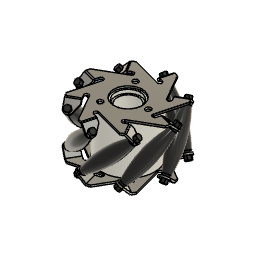
麦克纳姆轮A v5 (Autodesk Fusion 360 design; units mm, degrees)
Autodesk Fusion 360 part; units mm, degrees
note: some values were not read from the file. Set by a fixed rule: which sketch regions a step uses.
sketch "草图1" plane through (0, 0, 0) normal (0, 0, 1) x (1, 0, 0)
  circle A0 centre (0, 0) radius 8
  line L0 (-15.1925, 2.6566) -> (-15.1925, 19.6566)
  line L1 (-15.1925, 19.6566) -> (-10.2428, 14.7068)
  arc A1 (-10.2428, 14.7068) -> (-8.8643, 12.6212) centre (-9.5407, 13.6725) ccw
  line L2 (-12.6212, -8.8643) -> (-24.642, 3.1565)
  line L3 (-24.642, 3.1565) -> (-17.642, 3.1565)
  arc A2 (-17.642, 3.1565) -> (-15.1925, 2.6566) centre (-16.4142, 2.9216) ccw
  line L4 (-2.6566, -15.1925) -> (-19.6566, -15.1925)
  line L5 (-19.6566, -15.1925) -> (-14.7068, -10.2428)
  arc A3 (-14.7068, -10.2428) -> (-12.6212, -8.8643) centre (-13.6725, -9.5407) ccw
  line L6 (8.8643, -12.6212) -> (-3.1565, -24.642)
  line L7 (-3.1565, -24.642) -> (-3.1565, -17.642)
  arc A4 (-3.1565, -17.642) -> (-2.6566, -15.1925) centre (-2.9216, -16.4142) ccw
  line L8 (15.1925, -2.6566) -> (15.1925, -19.6566)
  line L9 (15.1925, -19.6566) -> (10.2428, -14.7068)
  arc A5 (10.2428, -14.7068) -> (8.8643, -12.6212) centre (9.5407, -13.6725) ccw
  line L10 (12.6212, 8.8643) -> (24.642, -3.1565)
  line L11 (24.642, -3.1565) -> (17.642, -3.1565)
  arc A6 (17.642, -3.1565) -> (15.1925, -2.6566) centre (16.4142, -2.9216) ccw
  line L12 (2.6566, 15.1925) -> (19.6566, 15.1925)
  line L13 (19.6566, 15.1925) -> (14.7068, 10.2428)
  arc A7 (14.7068, 10.2428) -> (12.6212, 8.8643) centre (13.6725, 9.5407) ccw
  line L14 (-8.8643, 12.6212) -> (3.1565, 24.642)
  line L15 (3.1565, 24.642) -> (3.1565, 17.642)
  arc A8 (3.1565, 17.642) -> (2.6566, 15.1925) centre (2.9216, 16.4142) ccw
  dimension "d1" = 16
  dimension "d2" = 2.5
  dimension "d3" = 45
  dimension "d4" = 7
  dimension "d5" = 17
  dimension "d7" = 360
  constraint coincident A0.centre origin
  constraint vertical L0
  constraint coincident L0 A2.end
  constraint coincident L12.start A8.end
  measures "d1" diameter of A0
  measures "d2" distance of L1.end A1.end
  measures "d3" angle of L0 L1
  measures "d4" distance of L0.end L1.end
  measures "d5" distance of L0.start L0.end
extrude "拉伸1" add sketch "草图1" along normal blind 1 makes body 1
sketch "草图2" plane through (0, 0, 1) normal (0, 0, 1) x (-1, 0, 0)
  circle A0 centre (0, 0) radius 8
  line L0 (-3.1565, -17.642) -> (-3.1565, -24.642)
  line L1 (-3.1565, -24.642) -> (8.8643, -12.6212)
  arc A1 (10.2428, -14.7068) -> (8.8643, -12.6212) centre (9.5407, -13.6725) ccw
  line L2 (10.2428, -14.7068) -> (15.1925, -19.6566)
  line L3 (15.1925, -19.6566) -> (15.1925, -2.6566)
  arc A2 (17.642, -3.1565) -> (15.1925, -2.6566) centre (16.4142, -2.9216) ccw
  line L4 (17.642, -3.1565) -> (24.642, -3.1565)
  line L5 (24.642, -3.1565) -> (12.6212, 8.8643)
  arc A3 (14.7068, 10.2428) -> (12.6212, 8.8643) centre (13.6725, 9.5407) ccw
  line L6 (14.7068, 10.2428) -> (19.6566, 15.1925)
  line L7 (19.6566, 15.1925) -> (2.6566, 15.1925)
  arc A4 (3.1565, 17.642) -> (2.6566, 15.1925) centre (2.9216, 16.4142) ccw
  line L8 (3.1565, 17.642) -> (3.1565, 24.642)
  line L9 (3.1565, 24.642) -> (-8.8643, 12.6212)
  arc A5 (-10.2428, 14.7068) -> (-8.8643, 12.6212) centre (-9.5407, 13.6725) ccw
  line L10 (-10.2428, 14.7068) -> (-15.1925, 19.6566)
  line L11 (-15.1925, 19.6566) -> (-15.1925, 2.6566)
  arc A6 (-17.642, 3.1565) -> (-15.1925, 2.6566) centre (-16.4142, 2.9216) ccw
  line L12 (-17.642, 3.1565) -> (-24.642, 3.1565)
  line L13 (-24.642, 3.1565) -> (-12.6212, -8.8643)
  arc A7 (-14.7068, -10.2428) -> (-12.6212, -8.8643) centre (-13.6725, -9.5407) ccw
  line L14 (-14.7068, -10.2428) -> (-19.6566, -15.1925)
  line L15 (-19.6566, -15.1925) -> (-2.6566, -15.1925)
  arc A8 (-3.1565, -17.642) -> (-2.6566, -15.1925) centre (-2.9216, -16.4142) ccw
  line L16 (3.1565, 17.642) -> (5.1565, 17.642)
  line L17 (5.1565, 17.642) -> (5.1565, 24.6526)
  line L18 (5.1565, 24.6526) -> (3.1565, 24.6526)
  line L19 (3.1565, 24.6526) -> (3.1565, 17.642)
  line L20 (-13.7858, 21.0782) -> (-15.2, 19.664)
  line L21 (-15.2, 19.664) -> (-10.2428, 14.7068)
  line L22 (-8.8286, 16.121) -> (-13.7858, 21.0782)
  line L23 (-10.2428, 14.7068) -> (-8.8286, 16.121)
  line L24 (-24.6526, 5.1565) -> (-24.6526, 3.1565)
  line L25 (-24.6526, 3.1565) -> (-17.642, 3.1565)
  line L26 (-17.642, 5.1565) -> (-24.6526, 5.1565)
  line L27 (-17.642, 3.1565) -> (-17.642, 5.1565)
  line L28 (-21.0782, -13.7858) -> (-19.664, -15.2)
  line L29 (-19.664, -15.2) -> (-14.7068, -10.2428)
  line L30 (-16.121, -8.8286) -> (-21.0782, -13.7858)
  line L31 (-14.7068, -10.2428) -> (-16.121, -8.8286)
  line L32 (-5.1565, -24.6526) -> (-3.1565, -24.6526)
  line L33 (-3.1565, -24.6526) -> (-3.1565, -17.642)
  line L34 (-5.1565, -17.642) -> (-5.1565, -24.6526)
  line L35 (-3.1565, -17.642) -> (-5.1565, -17.642)
  line L36 (13.7858, -21.0782) -> (15.2, -19.664)
  line L37 (15.2, -19.664) -> (10.2428, -14.7068)
  line L38 (8.8286, -16.121) -> (13.7858, -21.0782)
  line L39 (10.2428, -14.7068) -> (8.8286, -16.121)
  line L40 (24.6526, -5.1565) -> (24.6526, -3.1565)
  line L41 (24.6526, -3.1565) -> (17.642, -3.1565)
  line L42 (17.642, -5.1565) -> (24.6526, -5.1565)
  line L43 (17.642, -3.1565) -> (17.642, -5.1565)
  line L44 (21.0782, 13.7858) -> (19.664, 15.2)
  line L45 (19.664, 15.2) -> (14.7068, 10.2428)
  line L46 (16.121, 8.8286) -> (21.0782, 13.7858)
  line L47 (14.7068, 10.2428) -> (16.121, 8.8286)
  dimension "d10" = 2
  dimension "d12" = 360
  constraint horizontal L16
  constraint vertical L17
  constraint horizontal L18
  constraint vertical L19
  constraint coincident A4.start L8.start
  measures "d10" distance of L17.end L18.end
extrude "拉伸2" add sketch "草图2" against normal blind 1 contours L0 L32 L33 L34 L35 | L14 L28 L29 L30 L31 | L2 L36 L37 L38 L39 | L12 L24 L25 L26 L27 | L4 L40 L41 L42 L43 | L10 L20 L21 L22 L23 | L6 L44 L45 L46 L47 | L8 L16 L17 L18 L19 bodies 1
sketch "草图3" plane through (0, 0, 1) normal (0, 0, 1) x (-1, 0, 0)
  circle A0 centre (0, 0) radius 8
  line L0 (-3.1565, -24.642) -> (8.8643, -12.6212)
  arc A1 (10.2428, -14.7068) -> (8.8643, -12.6212) centre (9.5407, -13.6725) ccw
  line L1 (10.2428, -14.7068) -> (8.8286, -16.121)
  line L2 (8.8286, -16.121) -> (13.7858, -21.0782)
  line L3 (13.7858, -21.0782) -> (15.2, -19.664)
  line L4 (15.2, -19.664) -> (15.1925, -19.6566)
  line L5 (15.1925, -19.6566) -> (15.1925, -2.6566)
  arc A2 (17.642, -3.1565) -> (15.1925, -2.6566) centre (16.4142, -2.9216) ccw
  line L6 (17.642, -3.1565) -> (17.642, -5.1565)
  line L7 (17.642, -5.1565) -> (24.6526, -5.1565)
  line L8 (24.6526, -5.1565) -> (24.6526, -3.1565)
  line L9 (24.6526, -3.1565) -> (24.642, -3.1565)
  line L10 (24.642, -3.1565) -> (12.6212, 8.8643)
  arc A3 (14.7068, 10.2428) -> (12.6212, 8.8643) centre (13.6725, 9.5407) ccw
  line L11 (14.7068, 10.2428) -> (16.121, 8.8286)
  line L12 (16.121, 8.8286) -> (21.0782, 13.7858)
  line L13 (21.0782, 13.7858) -> (19.664, 15.2)
  line L14 (19.664, 15.2) -> (19.6566, 15.1925)
  line L15 (19.6566, 15.1925) -> (2.6566, 15.1925)
  arc A4 (3.1565, 17.642) -> (2.6566, 15.1925) centre (2.9216, 16.4142) ccw
  line L16 (3.1565, 17.642) -> (5.1565, 17.642)
  line L17 (5.1565, 17.642) -> (5.1565, 24.6526)
  line L18 (5.1565, 24.6526) -> (3.1565, 24.6526)
  line L19 (3.1565, 24.6526) -> (3.1565, 24.642)
  line L20 (3.1565, 24.642) -> (-8.8643, 12.6212)
  arc A5 (-10.2428, 14.7068) -> (-8.8643, 12.6212) centre (-9.5407, 13.6725) ccw
  line L21 (-10.2428, 14.7068) -> (-8.8286, 16.121)
  line L22 (-8.8286, 16.121) -> (-13.7858, 21.0782)
  line L23 (-13.7858, 21.0782) -> (-15.2, 19.664)
  line L24 (-15.2, 19.664) -> (-15.1925, 19.6566)
  line L25 (-15.1925, 19.6566) -> (-15.1925, 2.6566)
  arc A6 (-17.642, 3.1565) -> (-15.1925, 2.6566) centre (-16.4142, 2.9216) ccw
  line L26 (-17.642, 3.1565) -> (-17.642, 5.1565)
  line L27 (-17.642, 5.1565) -> (-24.6526, 5.1565)
  line L28 (-24.6526, 5.1565) -> (-24.6526, 3.1565)
  line L29 (-24.6526, 3.1565) -> (-24.642, 3.1565)
  line L30 (-24.642, 3.1565) -> (-12.6212, -8.8643)
  arc A7 (-14.7068, -10.2428) -> (-12.6212, -8.8643) centre (-13.6725, -9.5407) ccw
  line L31 (-14.7068, -10.2428) -> (-16.121, -8.8286)
  line L32 (-16.121, -8.8286) -> (-21.0782, -13.7858)
  line L33 (-21.0782, -13.7858) -> (-19.664, -15.2)
  line L34 (-19.664, -15.2) -> (-19.6566, -15.1925)
  line L35 (-19.6566, -15.1925) -> (-2.6566, -15.1925)
  arc A8 (-3.1565, -17.642) -> (-2.6566, -15.1925) centre (-2.9216, -16.4142) ccw
  line L36 (-3.1565, -17.642) -> (-5.1565, -17.642)
  line L37 (-5.1565, -17.642) -> (-5.1565, -24.6526)
  line L38 (-5.1565, -24.6526) -> (-3.1565, -24.6526)
  line L39 (-3.1565, -24.6526) -> (-3.1565, -24.642)
  circle A9 centre (0, 0) radius 11.5 construction
  line L40 (-14, 0) -> (17, 0)
  circle A10 centre (11.5, 0) radius 1.5
  circle A11 centre (-5.75, 9.9593) radius 1.5
  circle A12 centre (-5.75, -9.9593) radius 1.5
  dimension "d15" = 23
  dimension "d16" = 3
  dimension "d18" = 360
  constraint coincident A0.centre A9.centre
  constraint horizontal L40
  constraint coincident A9 A10.centre
  constraint coincident L40 A10.centre
  constraint coincident A0.centre L40
  measures "d15" diameter of A9
  measures "d16" diameter of A10
extrude "拉伸3" cut sketch "草图3" against normal blind 1 contours L40 A10 | L40 A10 | A11 | A12 bodies 1
sketch "草图4" plane through (-24.6526, 0, 0) normal (-1, 0, 0) x (0, -1, 0)
  line L0 (-3.1565, 1) -> (-5.1565, 1)
  line L1 (-5.1565, 1) -> (-5.1565, 0)
  line L2 (-5.1565, 0) -> (-3.1565, 0)
  line L3 (-3.1565, 0) -> (-3.1565, 1)
  line L4 (-3.1565, 0) -> (-5.1565, 0)
  line L5 (-5.1565, 0) -> (-5.1565, 1)
  line L6 (-12.9208, 0.5) -> (-0.2781, 0.5)
  line L7 (-10.8134, 5.2426) -> (-5.8636, 0.2929)
  arc A0 (-5.8636, 0.2929) -> (-5.1565, 0) centre (-5.0451, 1.2689) ccw
  line L8 (-5.1565, 1) -> (-10.1063, 5.9497)
  line L9 (-10.1063, 5.9497) -> (-10.8134, 5.2426)
  line L10 (-2.6566, 0) -> (-19.6566, 0)
  dimension "d82" = 1
  dimension "d83" = 7
  dimension "d84" = 7
  dimension "d85" = 45
  constraint coincident L2.end L3.start
  constraint coincident L1.end L2.start
  constraint coincident L0.end L1.start
  constraint symmetric L1.end L6 L0.end
  constraint symmetric L0.end L6 L1.end
  constraint perpendicular L7 L9
  constraint perpendicular L8 L9
  constraint parallel L6 L10
  measures "d82" distance of L7.start L8.end
  measures "d83" distance of L7.start L7.end
  measures "d84" distance of L0.end L8.end
  measures "d85" angle of L6 L8
extrude "拉伸4" add sketch "草图4" against normal blind 7 contours L0 L1 L3 L5 L6 bodies 1
extrude "拉伸17" add sketch "草图4" against normal blind 7 contours L1 L5 L6 L7 L8 L9 | L1 L5 L6 L7 A0 bodies 1
sketch "草图22" plane through (0, 2.0783, -2.0783) normal (0, -0.707107, 0.707107) x (1, 0, 0)
  line L0 (-24.6526, 11.3533) -> (-24.6526, 4.3533)
  line L1 (-24.6526, 4.3533) -> (-17.6526, 4.3533)
  line L2 (-17.6526, 4.3533) -> (-17.6526, 11.3533)
  line L3 (-17.6526, 11.3533) -> (-24.6526, 11.3533)
  line L4 (-17.6526, 6.3533) -> (-21.1526, 11.3533)
  dimension "d88" = 2
  constraint coincident L2 L4.start
  constraint midpoint L3 L4.end
  measures "d88" distance of L1.end L4.start
sketch "草图23" plane through (-19.4026, 8.3385, 4.182) normal (0, -0.707107, 0.707107) x (1, 0, 0)
extrude "拉伸18" cut sketch "草图22" against normal blind 1 contours L2 L3 L4 bodies 1
sketch "草图24" plane through (0, 2.0783, -2.0783) normal (0, -0.707107, 0.707107) x (1, 0, 0)
  line L0 (-17.6526, 6.3533) -> (-21.1526, 11.3533)
  line L1 (-21.1526, 11.3533) -> (-24.6526, 11.3533)
  line L2 (-24.6526, 11.3533) -> (-24.6526, 4.3533)
  line L3 (-24.6526, 4.3533) -> (-17.6526, 4.3533)
  line L4 (-17.6526, 4.3533) -> (-17.6526, 6.3533)
  line L5 (-20.4654, 10.3716) -> (-21.1526, 11.3533)
  line L6 (-24.6526, 11.3533) -> (-24.6526, 9.0517)
  arc A0 (-20.4654, 10.3716) -> (-24.6526, 9.0517) centre (-22.3509, 9.0517) ccw
  constraint tangent L0 A0
  constraint tangent L1 A0
  constraint tangent L2 A0
  constraint coincident L0.end L1.start
  constraint tangent L5 A0
  constraint coincident L1.end L2.start
  constraint coincident L2 L6.end
extrude "拉伸19" cut sketch "草图24" against normal blind 1 contours L0 L1 L5 A0 | L1 L2 L6 A0 bodies 1
sketch "草图25" plane through (0, 2.0783, -2.0783) normal (0, -0.707107, 0.707107) x (1, 0, 0)
  arc A0 (-20.4654, 10.3716) -> (-24.6526, 9.0517) centre (-22.3509, 9.0517) ccw
  line L0 (-24.6526, 9.0517) -> (-24.6526, 4.3533)
  line L1 (-24.6526, 4.3533) -> (-17.6526, 4.3533)
  line L2 (-17.6526, 4.3533) -> (-17.6526, 6.3533)
  line L3 (-17.6526, 6.3533) -> (-20.4654, 10.3716)
  circle A1 centre (-22.3509, 9.0517) radius 1.5
  dimension "d93" = 3
  constraint concentric A0 A1
  measures "d93" diameter of A1
extrude "拉伸20" cut sketch "草图25" against normal blind 1 contours A1 bodies 1
pattern_circular "C-阵列3" count 8 over 360 about axis through (0, 0, 1.75) along (0, 0, 1) of "拉伸17", "拉伸18", "拉伸19", "拉伸20"
copy_body "实体->零部件12" bodies 1 removing the originals makes body 2 in component "Component'"
sketch "草图26" plane through (0, 0, 0) normal (0, 0, 1) x (1, 0, 0)
  circle A0 centre (0, 0) radius 15
  dimension "d98" = 30
  constraint coincident A0.centre origin
  measures "d98" diameter of A0
extrude "拉伸21" add sketch "草图26" along normal blind 28 separate body makes body 3
sketch "草图27" plane through (0, 0, 28) normal (0, 0, 1) x (-1, 0, 0)
  circle A0 centre (0, 0) radius 15
  circle A1 centre (0, 0) radius 6
  dimension "d101" = 12
  constraint coincident A0.centre A1.centre
  measures "d101" diameter of A1
extrude "拉伸22" cut sketch "草图27" against normal blind 30 contours A1 bodies 3
sketch "草图28" plane through (0, 0, 28) normal (0, 0, 1) x (-1, 0, 0)
  circle A0 centre (0, 0) radius 6
  circle A1 centre (0, 0) radius 15
  circle A2 centre (0, 0) radius 7
  dimension "d104" = 14
  constraint coincident A0.centre A1.centre
  measures "d104" diameter of A2
extrude "拉伸23" cut sketch "草图28" against normal blind 2 contours A0 | A2 bodies 3
sketch "草图29" plane through (0, 0, 0) normal (0, 0, -1) x (1, 0, 0)
  circle A0 centre (0, 0) radius 6
  circle A1 centre (0, 0) radius 15
  circle A2 centre (0, 0) radius 7
  dimension "d107" = 14
  constraint concentric A0 A2
  measures "d107" diameter of A2
extrude "拉伸24" cut sketch "草图29" against normal blind 2 contours A0 | A2 bodies 3
sketch "草图30" plane through (0, 0, 28) normal (0, 0, 1) x (-1, 0, 0)
  circle A0 centre (0, 0) radius 7
  circle A1 centre (0, 0) radius 15
  circle A2 centre (0, 0) radius 11.5 construction
  line L0 (14, 0) -> (-14, 0)
  circle A3 centre (-11.5, 0) radius 1.5
  circle A4 centre (5.75, -9.9593) radius 1.5
  circle A5 centre (5.75, 9.9593) radius 1.5
  dimension "d110" = 23
  dimension "d111" = 3
  dimension "d113" = 360
  constraint coincident A0.centre A1.centre
  constraint horizontal L0
  constraint coincident A2 A3.centre
  constraint coincident L0 A3.centre
  constraint coincident A0.centre L0
  measures "d110" diameter of A2
  measures "d111" diameter of A3
extrude "拉伸25" cut sketch "草图30" against normal blind 30 contours L0 A3 | L0 A3 | A4 | A5 bodies 3
copy_body "实体->零部件13" bodies 3 removing the originals makes body 4 in component "Component''"
ref_plane "工作平面5" through (-22.2607, 1.3506, 3.3237) normal (0.183013, -0.683013, 0.707107) x (0.183013, -0.683013, -0.707107)
ref_plane "工作平面6" through (-14.7856, -16.6957, 24.6763) normal (-0.353553, 0.612372, -0.707107) x (-0.353553, 0.612372, 0.707107)
sketch "草图31" plane through (-14.7856, -16.6957, 24.6763) normal (-0.353553, 0.612372, -0.707107) x (-0.353553, 0.612372, 0.707107)
  circle A0 centre (-0.9979, -1.1984) radius 1.5
  arc A1 (-2.3178, 0.6872) -> (-0.9979, -3.5) centre (-0.9979, -1.1984) ccw
  line L0 (-0.9979, -3.5) -> (3.7005, -3.5)
  line L1 (3.7005, -3.5) -> (3.7005, 3.5)
  line L2 (3.7005, 3.5) -> (1.7005, 3.5)
  line L3 (1.7005, 3.5) -> (-2.3178, 0.6872)
  circle A2 centre (-0.9979, -1.1984) radius 2
  dimension "d126" = 4
  constraint concentric A0 A2
  measures "d126" diameter of A2
sketch "草图32" plane through (-22.2607, 1.3506, 3.3237) normal (0.183013, -0.683013, 0.707107) x (0.183013, -0.683013, -0.707107)
  circle A0 centre (-0.9979, -1.1984) radius 1.5
  arc A1 (-2.3178, 0.6872) -> (-0.9979, -3.5) centre (-0.9979, -1.1984) ccw
  line L0 (-0.9979, -3.5) -> (3.7005, -3.5)
  line L1 (3.7005, -3.5) -> (3.7005, 3.5)
  line L2 (3.7005, 3.5) -> (1.7005, 3.5)
  line L3 (1.7005, 3.5) -> (-2.3178, 0.6872)
  circle A2 centre (-0.9979, -1.1984) radius 2
  dimension "d127" = 4
  constraint concentric A0 A2
  measures "d127" diameter of A2
ref_plane "工作平面7" through (-18.983, -8.3097, 13.5908) normal (0.269433, -0.650469, 0.710138) x (0.184952, -0.688729, -0.701032)
sketch "草图33" plane through (-18.983, -8.3097, 13.5908) normal (0.269433, -0.650469, 0.710138) x (0.184952, -0.688729, -0.701032)
  circle A0 centre (-0.5, -0.5) radius 4
  dimension "d128" = 8
  measures "d128" diameter of A0
loft "放样2" add profiles "草图32", "草图33", "草图31" section 1 contours A2 section 2 section 3 contours A2 separate body makes body 5
sketch "草图34" plane through (-0.4843, 1.8074, -1.8712) normal (-0.183013, 0.683013, -0.707107) x (-0.965926, -0.258819, 0)
  circle A0 centre (22.3509, 8.3446) radius 2
  circle A1 centre (22.3509, 8.3446) radius 1.5
  dimension "d129" = 3
  constraint concentric A0 A1
  measures "d129" diameter of A1
extrude "拉伸26" add sketch "草图34" along normal blind 4 contours A1 bodies 5
sketch "草图35" plane through (7.9356, -13.7448, 15.8712) normal (0.353553, -0.612372, 0.707107) x (0.866025, 0.5, 0)
  circle A0 centre (-22.3509, 11.4544) radius 2
  circle A1 centre (-22.3509, 11.4544) radius 1.5
  dimension "d132" = 3
  constraint concentric A0 A1
  measures "d132" diameter of A1
extrude "拉伸27" add sketch "草图35" along normal blind 4 contours A1 bodies 5
sketch "草图36" plane through (9.3498, -16.1943, 18.6996) normal (0.353553, -0.612372, 0.707107) x (0.866025, 0.5, 0)
  circle A0 centre (-22.3509, 11.4544) radius 1.5
  line L0 (-24.0625, 11.7202) -> (-23.4369, 10.1051)
  line L1 (-23.4369, 10.1051) -> (-21.7253, 9.8393)
  line L2 (-21.7253, 9.8393) -> (-20.6394, 11.1886)
  line L3 (-20.6394, 11.1886) -> (-21.265, 12.8038)
  line L4 (-21.265, 12.8038) -> (-22.9766, 13.0695)
  line L5 (-22.9766, 13.0695) -> (-24.0625, 11.7202)
  point P0 (-22.3509, 11.4544)
  constraint coincident P0 A0.centre
extrude "拉伸28" add sketch "草图36" against normal blind 2 contours A0 L2 L3 | A0 L3 L4 | A0 L1 L2 | A0 L4 L5 | A0 L0 L1 | A0 L0 L5 bodies 5
sketch "草图37" plane through (-1.2163, 4.5395, -4.6996) normal (-0.183013, 0.683013, -0.707107) x (-0.965926, -0.258819, 0)
  circle A0 centre (22.3509, 8.3446) radius 1.5
  line L0 (24.0787, 8.2221) -> (23.3209, 9.7796)
  line L1 (23.3209, 9.7796) -> (21.5932, 9.9021)
  line L2 (21.5932, 9.9021) -> (20.6232, 8.4671)
  line L3 (20.6232, 8.4671) -> (21.381, 6.9096)
  line L4 (21.381, 6.9096) -> (23.1087, 6.7871)
  line L5 (23.1087, 6.7871) -> (24.0787, 8.2221)
  point P0 (22.3509, 8.3446)
  constraint coincident P0 A0.centre
extrude "拉伸29" add sketch "草图37" against normal blind 2 contours A0 L0 L5 | A0 L0 L1 | A0 L4 L5 | A0 L1 L2 | A0 L3 L4 | A0 L2 L3 bodies 5
pattern_circular "C-阵列4" count 8 over 360 about axis through (0, 0, 1.75) along (0, 0, 1) of bodies 5 makes body 6 at (-6.2668, -17.3337, 10.8202) makes body 7 at (7.8255, -16.6881, 10.8202) makes body 8 at (17.3337, -6.2668, 10.8202) makes body 9 at (16.6881, 7.8255, 10.8202) makes body 10 at (6.2668, 17.3337, 10.8202) makes body 11 at (-7.8255, 16.6881, 10.8202) makes body 12 at (-17.3337, 6.2668, 10.8202)
copy_body "实体->零部件14" bodies 5 removing the originals makes body 13 in component "Component'''"
copy_body "实体->零部件15" bodies 6 removing the originals makes body 14 in component "Component''''"
copy_body "实体->零部件16" bodies 7 removing the originals makes body 15 in component "Component'''''"
copy_body "实体->零部件17" bodies 8 removing the originals makes body 16 in component "Component''''''"
copy_body "实体->零部件18" bodies 9 removing the originals makes body 17 in component "Component'''''''"
copy_body "实体->零部件19" bodies 10 removing the originals makes body 18 in component "Component''''''''"
copy_body "实体->零部件20" bodies 11 removing the originals makes body 19 in component "Component'''''''''"
copy_body "实体->零部件21" bodies 12 removing the originals makes body 20 in component "Component''''''''''"
component "Component'" placed x (0.5, 0.866025, 0) y (-0.866025, 0.5, 0) z (0, 0, 1) at (0, 0, -1)
component "Component''" placed x (1, 0, 0) y (0, 1, 0) z (0, 0, 1) at (0, 0, 0)
component "Component'" placed x (0.5, -0.866025, 0) y (-0.866025, -0.5, 0) z (0, 0, -1) at (0, 0, 29)
component "Component'''" placed x (1, 0, 0) y (0, 1, 0) z (0, 0, 1) at (0, 0, 0)
component "Component''''" placed x (1, 0, 0) y (0, 1, 0) z (0, 0, 1) at (0, 0, 0)
component "Component'''''" placed x (1, 0, 0) y (0, 1, 0) z (0, 0, 1) at (0, 0, 0)
component "Component''''''" placed x (1, 0, 0) y (0, 1, 0) z (0, 0, 1) at (0, 0, 0)
component "Component'''''''" placed x (1, 0, 0) y (0, 1, 0) z (0, 0, 1) at (0, 0, 0)
component "Component''''''''" placed x (1, 0, 0) y (0, 1, 0) z (0, 0, 1) at (0, 0, 0)
component "Component'''''''''" placed x (1, 0, 0) y (0, 1, 0) z (0, 0, 1) at (0, 0, 0)
component "Component''''''''''" placed x (1, 0, 0) y (0, 1, 0) z (0, 0, 1) at (0, 0, 0)
